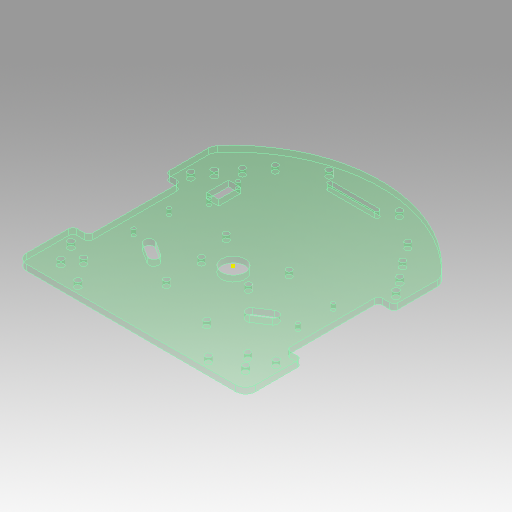
# Autodesk Inventor part: base_chasis_v6
Saved by Autodesk Inventor 2027 (Build 310192000, 192)
## iProperties
Created: 2025-03-12
Part Number: base_chasis_v6
Material: Generic
Document SubType Name: Modeling
Designer: cdavi
Density: 1 g/cm^3
Appearance: Clear - Green 1
Author: cdavi
Autodesk Inventor part; units mm, degrees
ref_plane "YZ Plane" through (0, 0, 0) normal (1, 0, 0) x (0, 1, 0)
ref_plane "XZ Plane" through (0, 0, 0) normal (0, 1, 0) x (-1, 0, 0)
ref_plane "XY Plane" through (0, 0, 0) normal (0, 0, 1) x (1, 0, 0)
sketch "Sketch1" plane through (0, 0, 0) normal (0, 1, 0) x (-1, 0, 0)
  line L0 (50.9902, 55) -> (-50.9902, 55)
  line L1 (12, -62.25) -> (-12, -62.25)
  line L2 (-12, -60) -> (12, -60)
  circle A0 centre (0, 0) radius 6
  circle A1 centre (-44.3523, -52.8571) radius 1.5 construction
  circle A2 centre (-41.7906, 34.5) radius 1.5
  circle A3 centre (-20, 51.5) radius 1.5 construction
  circle A4 centre (41.7906, 34.5) radius 1.5
  circle A5 centre (20, 51.5) radius 1.5 construction
  circle A6 centre (44.3523, -52.8571) radius 1.5 construction
  arc A7 (12, -62.25) -> (12, -60) centre (12, -61.125) ccw
  arc A8 (-12, -60) -> (-12, -62.25) centre (-12, -61.125) ccw
  circle A9 centre (0, 0) radius 69 construction
  line L3 (0, 0) -> (0, 55)
  arc A10 (-50.9902, 55) -> (50.9902, 55) centre (0, 0) ccw
  line L4 (0, 0) -> (-75, 0)
  line L5 (0, 0) -> (62.5352, -29.1607) construction
  line L6 (0, 0) -> (69, 0)
  line L7 (0, 0) -> (41.7906, 34.5) construction
  line L8 (50.2232, 23.5) -> (71.2232, 23.5)
  line L9 (71.2232, 23.5) -> (71.2232, -23.5)
  line L10 (71.2232, -23.5) -> (50.2232, -23.5)
  line L11 (50.2232, -23.5) -> (50.2232, 23.5)
  line L12 (50.2232, 23.5) -> (71.2232, -23.5) construction
  line L13 (71.2232, 23.5) -> (50.2232, -23.5) construction
  circle A11 centre (41.8232, -9) radius 1
  circle A12 centre (41.8232, 9) radius 1
  circle A13 centre (16, -12.35) radius 1.5
  circle A14 centre (33.75, -55) radius 1.5
  circle A15 centre (-16, -12.35) radius 1.5
  circle A16 centre (-33.75, -55) radius 1.5
  line L14 (-50.2232, 23.5) -> (-71.2232, 23.5)
  line L15 (-71.2232, 23.5) -> (-71.2232, -23.5)
  line L16 (-71.2232, -23.5) -> (-50.2232, -23.5)
  line L17 (-50.2232, -23.5) -> (-50.2232, 23.5)
  circle A17 centre (-41.8232, -9) radius 1
  circle A18 centre (-41.8232, 9) radius 1
  line L18 (39, -25.5) -> (33, -25.5)
  line L19 (33, -25.5) -> (33, -36.5)
  line L20 (33, -36.5) -> (39, -36.5)
  line L21 (39, -36.5) -> (39, -25.5)
  circle A19 centre (36, -38.5) radius 1
  line L22 (39, -31) -> (33, -31)
  circle A20 centre (36, -23.5) radius 1
  circle A21 centre (40.817, -45.3318) radius 1.5
  circle A22 centre (-41.7906, 34.5) radius 1.5
  circle A23 centre (-40.817, -45.3318) radius 1.5
  line L23 (41.7906, 34.5) -> (41.7906, 39.5)
  line L24 (41.7906, 39.5) -> (63.7554, 39.5) construction
  line L25 (0, 0) -> (44.3523, -52.8571) construction
  line L26 (40.817, -45.3318) -> (0, 0) construction
  line L27 (0, 0) -> (62.5352, 29.1607) construction
  circle A24 centre (12, 4.32) radius 1.5
  circle A25 centre (-12, 4.32) radius 1.5
  line L28 (33.2906, 29.5) -> (34.2906, 29.5)
  line L29 (36.2906, 27.5) -> (36.2906, 21.5)
  line L30 (34.2906, 19.5) -> (33.2906, 19.5)
  line L31 (31.2906, 21.5) -> (31.2906, 27.5)
  arc A26 (34.2906, 19.5) -> (36.2906, 21.5) centre (34.2906, 21.5) ccw
  arc A27 (31.2906, 21.5) -> (33.2906, 19.5) centre (33.2906, 21.5) ccw
  arc A28 (33.2906, 29.5) -> (31.2906, 27.5) centre (33.2906, 27.5) ccw
  arc A29 (36.2906, 27.5) -> (34.2906, 29.5) centre (34.2906, 27.5) ccw
  line L32 (0, 0) -> (-41.7906, 34.5) construction
  line L33 (-33.2906, 29.5) -> (-34.2906, 29.5)
  line L34 (-36.2906, 27.5) -> (-36.2906, 21.5)
  line L35 (-34.2906, 19.5) -> (-33.2906, 19.5)
  line L36 (-31.2906, 21.5) -> (-31.2906, 27.5)
  arc A30 (-36.2906, 21.5) -> (-34.2906, 19.5) centre (-34.2906, 21.5) ccw
  arc A31 (-33.2906, 19.5) -> (-31.2906, 21.5) centre (-33.2906, 21.5) ccw
  arc A32 (-31.2906, 27.5) -> (-33.2906, 29.5) centre (-33.2906, 27.5) ccw
  arc A33 (-34.2906, 29.5) -> (-36.2906, 27.5) centre (-34.2906, 27.5) ccw
  circle A34 centre (0, 0) radius 54.1913
  circle A35 centre (0, 0) radius 61 construction
  point P0 (-5.9883, -61.0615)
  point P1 (60.7232, 0)
  point P2 (0, 34.5)
  point P3 (36, -36.5)
  point P4 (50.9902, 55)
  point P5 (0, -6)
  point P6 (31.2906, 29.5)
  point P7 (31.2906, 19.5)
  point P8 (33.7906, 29.5)
  point P9 (-31.2906, 29.5)
  point P10 (-31.2906, 19.5)
  point P11 (-33.7906, 29.5)
  dimension "d12" = 12
  dimension "d287" = 0
  dimension "d398" = 108.3827
  dimension "d0" = 3
  dimension "d1" = 3
  dimension "d15" = 24
  dimension "d16" = 3
  dimension "d62" = 2.25
  dimension "d148" = 3.5
  dimension "d276" = 138
  dimension "d285" = 150
  dimension "d286" = 55
  dimension "d288" = 12
  dimension "d289" = 40
  dimension "d290" = 3.5
  dimension "d291" = 20
  dimension "d293" = 25
  dimension "d300" = 21
  dimension "d301" = 47
  dimension "d304" = 2
  dimension "d305" = 8.4
  dimension "d306" = 9
  dimension "d307" = 3
  dimension "d311" = 16
  dimension "d318" = 33.75
  dimension "d323" = 11
  dimension "d324" = 6
  dimension "d325" = 2
  dimension "d326" = 2
  dimension "d327" = 15
  dimension "d338" = 33
  dimension "d342" = 5
  dimension "d345" = 11
  dimension "d346" = 39.541
  dimension "d348" = 40
  dimension "d350" = 61
  dimension "d351" = 48
  dimension "d352" = 3
  dimension "d353" = 12.35
  dimension "d354" = 55
  dimension "d355" = 25
  dimension "d356" = 60
  dimension "d358" = 71.2232
  dimension "d371" = 3
  dimension "d372" = 12
  dimension "d373" = 4.32
  dimension "d393" = 5
  dimension "d394" = 10
  dimension "d395" = 5
  dimension "d396" = 2
  dimension "d397" = 8
  constraints: 75 end point, 33 centre point, 30 point on circle, 29 symmetric about line, 11 point on line, 11 tangent, 9 horizontal, 8 coincident, 8 midpoint, 7 parallel, 5 equal radius, 5 perpendicular, 3 vertical, 3 vertical alignment, 1 horizontal alignment, 33 other
  measures "d0" diameter of A4
  measures "d1" diameter of A5
  measures "d15" distance of L1.end L1.start
  measures "d16" diameter of A6
  measures "d62" distance between parallel lines of L1 L2
  measures "d148" distance from line of L0 A5.centre
  measures "d276" diameter of A9
  measures "d285" diameter of A10
  measures "d286" distance from line of L0 point (0, 0)
  measures "d288" horizontal distance of point (0, 0) A7.centre
  measures "d289" distance of A5.centre A3.centre
  measures "d290" distance from line of L0 A3.centre
  measures "d291" distance from line of L3 A5.centre
  measures "d293" angle of L6 L5
  measures "d300" distance of L9.end L10.end
  measures "d301" distance of L10.end L8.start
  measures "d304" diameter of A11
  measures "d305" distance from line of L11 A11.centre
  measures "d306" distance from line of L6 A11.centre
  measures "d307" diameter of A13
  measures "d311" horizontal distance of point (0, 0) A13.centre
  measures "d318" distance from line of L3 A14.centre
  measures "d323" distance of L18.end L19.end
  measures "d324" distance of L18.start L18.end
  measures "d325" distance from line of L10.end L18
  measures "d326" diameter of A19
  measures "d327" distance of A20.centre A19.centre
  measures "d338" distance between parallel lines of L3 L19
  measures "d342" distance of L7.end L23.end
  measures "d345" distance from line of L8 L7.end
  measures "d346" angle of L6 L7
  measures "d348" angle of L3 L25
  measures "d350" distance of L26.start L4.start
  measures "d351" angle of L6 L26
  measures "d352" diameter of A21
  measures "d353" vertical distance of point (0, 0) A13.centre
  measures "d354" distance from line of L6 A14.centre
  measures "d355" angle of L27 L6
  measures "d356" distance between parallel lines of L2 L4
  measures "d358" distance between parallel lines of L3 L15
  measures "d371" diameter of A24
  measures "d372" horizontal distance of A24.centre point (0, 0)
  measures "d373" vertical distance of point (0, 0) A24.centre
  measures "d393" distance between parallel lines of L31 L29
  measures "d394" distance of point (31.291, 19.5) point (31.291, 29.5)
  measures "d395" distance from line of L7.end L28
  measures "d396" radius of A26
  measures "d397" horizontal distance of L7.end point (33.791, 29.5)
extrude "Extrusion1" add sketch "Sketch1" along normal blind 3 contours A10 L8 L11 A34 A4 L3 L0 | L3 A34 A2 L17 L14 A10 L0 | A34 A4 L11 L6 A0 L3 | L3 A0 L4 L17 A34 A2 | A10 L16 L17 A34 L11 L10 | L6 L11 A34 L17 L4 A0
sketch "Sketch3" plane through (0, 3, 0) normal (0, 1, 0) x (1, 0, 0)
  line L0 (3, 0) -> (3, -20)
  circle A0 centre (-11, -23.1) radius 1.5
  line L1 (-50.9902, -55) -> (50.9902, -55) projected
  circle A1 centre (17, -30.6) radius 1.5
  point P0 (0, 0)
  point P1 (-51.2348, -50)
  dimension "d377" = 20
  dimension "d378" = 3
  dimension "d379" = 3
  dimension "d380" = 14
  dimension "d381" = 31.9
  dimension "d383" = 14
  dimension "d384" = 3
  dimension "d385" = 24.4
  constraints: 2 centre point, 2 end point, 1 vertical, 1 other
  measures "d377" distance of L0.start L0.end
  measures "d378" distance from line of point (0, 0) L0
  measures "d379" diameter of A0
  measures "d380" distance from line of L0 A0.centre
  measures "d383" distance from line of A1.centre L0
  measures "d384" diameter of A1
fillet "Fillet1" radius 2 1 edges at (71.2232, 1.5, 23.5)
fillet "Fillet2" radius 2 7 edges at (71.2232, 1.5, -23.5) (-71.2232, 1.5, -23.5) (-71.2232, 1.5, 23.5) (-50.2232, 1.5, -23.5) (-50.2232, 1.5, 23.5) (50.2232, 1.5, -23.5) (50.2232, 1.5, 23.5)
hole "Hole1" at (-11, 3, 23.1) at (17, 3, 30.6) direction (0, -1, 0) diameter 3 end through all
sketch "Sketch4" plane through (0, 3, 0) normal (0, 1, 0) x (1, 0, 0)
  line L0 (-50.2232, 21.5) -> (-50.2232, -21.5) projected
  line L1 (-115.8769, 106.6342) -> (-58.2232, 106.6342)
  line L2 (-58.2232, 106.6342) -> (-58.2232, -77.5521)
  line L3 (-58.2232, -77.5521) -> (-115.8769, -77.5521)
  line L4 (-115.8769, -77.5521) -> (-115.8769, 106.6342)
  line L5 (-50.2232, 0) -> (-58.2232, 0)
  point P0 (0, 0)
  dimension "d403" = 8
  constraints: 10 end point, 2 parallel, 2 perpendicular, 1 horizontal, 1 midpoint, 1 point on line
  measures "d403" distance of L5.start L5.end
extrude "Extrusion3" cut sketch "Sketch4" against normal blind 10
mirror "Mirror1" about plane through (0, 0, 0) normal (1, 0, 0) of "Extrusion3"
fillet "Fillet3" radius 2 4 edges at (-58.2232, 1.5, 23.5) (-58.2232, 1.5, -23.5) (58.2232, 1.5, -23.5) (58.2232, 1.5, 23.5)
sketch "Sketch5" plane through (0, 3, 0) normal (0, 1, 0) x (1, 0, 0)
  point P0 (0, 0)
fillet "Fillet5" [suppressed]
sketch "Sketch6" plane through (0, 3, 0) normal (0, 1, 0) x (1, 0, 0)
  point P0 (0, 0)
sketch "Sketch7" plane through (0, 3, 0) normal (0, 1, 0) x (1, 0, 0)
  arc A0 (58.2232, 47.2764) -> (-58.2232, 47.2764) centre (0, 0) ccw projected
  line L0 (-58.2232, 47.2764) -> (-58.2232, 0)
  line L1 (-58.2232, 0) -> (0, 0)
  line L2 (-58.2232, 0) -> (-58.2232, 23.5)
  line L3 (-56.2232, 23.5) -> (-52.2232, 23.5) projected
  constraints: 6 end point, 1 horizontal, 1 perpendicular, 1 point on line, 1 vertical
sketch "Sketch8" plane through (0, 3, 0) normal (0, 1, 0) x (1, 0, 0)
  line L0 (58.2232, 47.2764) -> (58.2232, 25.5) projected
  line L1 (58.2232, 47.2764) -> (58.2232, 23)
  point P0 (0, 0)
  constraints: 2 end point, 1 vertical
fillet "Fillet6" radius 5 2 edges at (-58.2232, 1.5, -47.2764) (58.2232, 1.5, -47.2764)
sketch "Sketch9" plane through (0, 3, 0) normal (0, 1, 0) x (1, 0, 0)
  arc A0 (50.9902, -55) -> (58.2232, -47.2764) centre (0, 0) ccw projected
  line L0 (50.9902, -55) -> (58.2232, -55)
  line L1 (58.2232, -55) -> (58.2232, -47.2764)
  circle A1 centre (0, 0) radius 6 projected
  arc A2 (50.9902, -55) -> (58.2232, -47.2764) centre (0, 0) ccw
  constraints: 4 end point, 2 point on circle, 1 centre point, 1 coincident, 1 horizontal, 1 perpendicular
extrude "Extrusion4" add sketch "Sketch9" against normal blind 3 contours A0 L1 L0
mirror "Mirror2" about plane through (0, 0, 0) normal (1, 0, 0) of "Extrusion4"
sketch "Sketch10" plane through (0, 3, 0) normal (0, 1, 0) x (1, 0, 0)
  point P0 (0, 0)
sketch "Sketch11" plane through (0, 3, 0) normal (0, 1, 0) x (1, 0, 0)
  line L0 (-58.2232, -55) -> (58.2232, -55) projected
  line L1 (58.2232, -25.5) -> (58.2232, -55) projected
  line L2 (-58.2232, -55) -> (58.2232, -55)
  line L3 (58.2232, -55) -> (58.2232, -52)
  line L4 (58.2232, -52) -> (-58.2232, -52)
  line L5 (-58.2232, -52) -> (-58.2232, -55)
  point P0 (0, 0)
  dimension "d410" = 3
  constraints: 8 end point, 2 parallel, 1 horizontal, 1 perpendicular, 1 point on line
  measures "d410" distance between parallel lines of L0 L4
extrude "Extrusion5" cut sketch "Sketch11" against normal blind 3
fillet "Fillet7" radius 5 2 edges at (58.2232, 1.5, 52) (-58.2232, 1.5, 52)
sketch "Sketch12" plane through (0, 3, 0) normal (0, 1, 0) x (1, 0, 0)
  point P0 (0, 0)
sketch "Sketch13" plane through (0, 3, 0) normal (0, 1, 0) x (1, 0, 0)
  circle A0 centre (-33.2232, -46) radius 1.6
  line L0 (-53.2232, -52) -> (53.2232, -52) projected
  line L1 (-58.2232, -47) -> (-58.2232, -25.5) projected
  line L2 (53.2232, -52) -> (-53.2232, -52) projected
  line L3 (0, -52) -> (0, 75)
  arc A1 (57.0249, 48.7151) -> (-57.0249, 48.7151) centre (0, 0) ccw projected
  circle A2 centre (-52.2232, -30.525) radius 1.6
  line L4 (0, 0) -> (-64.2535, 0)
  line L5 (0, 0) -> (-17.8585, 66.6489)
  circle A3 centre (0, 0) radius 69
  circle A4 centre (0, 0) radius 6 projected
  circle A5 centre (-17.8585, 66.6489) radius 1.6
  circle A6 centre (33.2232, -46) radius 1.6
  circle A7 centre (52.2232, -30.525) radius 1.6
  circle A8 centre (17.8585, 66.6489) radius 1.6
  line L6 (-58.2232, 45.4674) -> (-58.2232, 25.5) projected
  line L7 (-56.2232, 23.5) -> (-52.2232, 23.5) projected
  circle A9 centre (-52.2232, 30.525) radius 1.6
  circle A10 centre (52.2232, 30.525) radius 1.6
  circle A11 centre (-47.2235, 37.4674) radius 1.6
  circle A12 centre (-47.0232, -40.8) radius 1.6
  circle A13 centre (47.2235, 37.4674) radius 1.6
  circle A14 centre (47.0232, -40.8) radius 1.6
  line L8 (-52.2232, -23.5) -> (-56.2232, -23.5) projected
  point P0 (-54.2232, 23.5)
  dimension "d414" = 3.2
  dimension "d415" = 6
  dimension "d416" = 25
  dimension "d417" = 3.2
  dimension "d418" = 6
  dimension "d420" = 75
  dimension "d421" = 6
  dimension "d422" = 3.2
  dimension "d427" = 3.2
  dimension "d428" = 6
  dimension "d429" = 7.025
  dimension "d430" = 3.2
  dimension "d432" = 10.9998
  dimension "d433" = 3.2
  dimension "d434" = 11.2
  dimension "d435" = 11.2
  dimension "d436" = 13.9674
  dimension "d437" = 7.025
  constraints: 12 centre point, 6 end point, 6 symmetric about line, 2 midpoint, 1 coincident, 1 horizontal, 1 point on circle, 1 point on line, 1 vertical, 10 other
  measures "d414" diameter of A0
  measures "d415" distance from line of L0 A0.centre
  measures "d416" distance from line of L1 A0.centre
  measures "d417" diameter of A2
  measures "d418" distance from line of L1 A2.centre
  measures "d420" angle of L4 L5
  measures "d422" diameter of A5
  measures "d427" diameter of A9
  measures "d428" distance from line of L6 A9.centre
  measures "d429" distance from line of L7 A9.centre
  measures "d430" diameter of A11
  measures "d432" distance from line of L6 A11.centre
  measures "d433" diameter of A12
  measures "d434" distance from line of L2 A12.centre
  measures "d435" distance from line of L1 A12.centre
  measures "d436" distance from line of L7 A11.centre
  measures "d437" distance from line of L8 A2.centre
extrude "Extrusion6" cut sketch "Sketch13" against normal blind 3 contours A0 | A5 A3 | A3 L5 A5 | A8 A3 | A3 A8 | A3 A5 L5 | A2 | A6 | A7 | A9 | A10 | A11 | A12 | A13 | A14
sketch "Sketch14" plane through (0, 0, 0) normal (0, -1, 0) x (1, 0, 0)
  circle A0 centre (47.2235, -37.4674) radius 1.6 projected
  circle A1 centre (-52.2232, 30.525) radius 1.6 projected
  circle A2 centre (17.8585, -66.6489) radius 1.6 projected
  circle A3 centre (52.2232, 30.525) radius 1.6 projected
  circle A4 centre (52.2232, -30.525) radius 1.6 projected
  circle A5 centre (-47.2235, -37.4674) radius 1.6 projected
  circle A6 centre (47.0232, 40.8) radius 1.6 projected
  circle A7 centre (-33.2232, 46) radius 1.6 projected
  circle A8 centre (-17.8585, -66.6489) radius 1.6 projected
  circle A9 centre (33.2232, 46) radius 1.6 projected
  circle A10 centre (-52.2232, -30.525) radius 1.6 projected
  circle A11 centre (-47.0232, 40.8) radius 1.6 projected
  arc A12 (-53.2232, 52) -> (-58.2232, 47) centre (-53.2232, 47) ccw projected
  line L0 (-53.2232, 52) -> (53.2232, 52) projected
  arc A13 (58.2232, 47) -> (53.2232, 52) centre (53.2232, 47) ccw projected
  line L1 (58.2232, 47) -> (58.2232, 25.5) projected
  arc A14 (56.2232, 23.5) -> (58.2232, 25.5) centre (56.2232, 25.5) ccw projected
  line L2 (56.2232, 23.5) -> (52.2232, 23.5) projected
  arc A15 (52.2232, 23.5) -> (50.2232, 21.5) centre (52.2232, 21.5) ccw projected
  line L3 (50.2232, 21.5) -> (50.2232, -21.5) projected
  arc A16 (50.2232, -21.5) -> (52.2232, -23.5) centre (52.2232, -21.5) ccw projected
  line L4 (52.2232, -23.5) -> (56.2232, -23.5) projected
  arc A17 (58.2232, -25.5) -> (56.2232, -23.5) centre (56.2232, -25.5) ccw projected
  line L5 (58.2232, -25.5) -> (58.2232, -45.4674) projected
  arc A18 (57.0249, -48.7151) -> (58.2232, -45.4674) centre (53.2232, -45.4674) ccw projected
  arc A19 (-57.0249, -48.7151) -> (57.0249, -48.7151) centre (0, 0) ccw projected
  arc A20 (-58.2232, -45.4674) -> (-57.0249, -48.7151) centre (-53.2232, -45.4674) ccw projected
  line L6 (-58.2232, -45.4674) -> (-58.2232, -25.5) projected
  arc A21 (-56.2232, -23.5) -> (-58.2232, -25.5) centre (-56.2232, -25.5) ccw projected
  line L7 (-56.2232, -23.5) -> (-52.2232, -23.5) projected
  arc A22 (-52.2232, -23.5) -> (-50.2232, -21.5) centre (-52.2232, -21.5) ccw projected
  line L8 (-50.2232, -21.5) -> (-50.2232, 21.5) projected
  arc A23 (-50.2232, 21.5) -> (-52.2232, 23.5) centre (-52.2232, 21.5) ccw projected
  line L9 (-52.2232, 23.5) -> (-56.2232, 23.5) projected
  arc A24 (-58.2232, 25.5) -> (-56.2232, 23.5) centre (-56.2232, 25.5) ccw projected
  line L10 (-58.2232, 25.5) -> (-58.2232, 47) projected
  circle A25 centre (17, 30.6) radius 1.5 projected
  circle A26 centre (-11, 23.1) radius 1.5 projected
  circle A27 centre (0, 0) radius 6 projected
  line L11 (12, -60) -> (-12, -60) projected
  arc A28 (-12, -60) -> (-12, -62.25) centre (-12, -61.125) ccw projected
  line L12 (-12, -62.25) -> (12, -62.25) projected
  arc A29 (12, -62.25) -> (12, -60) centre (12, -61.125) ccw projected
  circle A30 centre (-41.8232, -9) radius 1 projected
  circle A31 centre (-16, -12.35) radius 1.5 projected
  circle A32 centre (-33.75, -55) radius 1.5 projected
  circle A33 centre (16, -12.35) radius 1.5 projected
  circle A34 centre (33.75, -55) radius 1.5 projected
  circle A35 centre (41.8232, -9) radius 1 projected
  circle A36 centre (-36, -38.5) radius 1 projected
  circle A37 centre (-36, -23.5) radius 1 projected
  circle A38 centre (-40.817, -45.3318) radius 1.5 projected
  circle A39 centre (40.817, -45.3318) radius 1.5 projected
  line L13 (-33, -25.5) -> (-39, -25.5) projected
  line L14 (-39, -25.5) -> (-39, -36.5) projected
  line L15 (-39, -36.5) -> (-33, -36.5) projected
  line L16 (-33, -36.5) -> (-33, -25.5) projected
  circle A40 centre (41.8232, 9) radius 1 projected
  circle A41 centre (12, 4.32) radius 1.5 projected
  arc A42 (34.2906, 19.5) -> (36.2906, 21.5) centre (34.2906, 21.5) ccw projected
  line L17 (36.2906, 21.5) -> (36.2906, 27.5) projected
  arc A43 (36.2906, 27.5) -> (34.2906, 29.5) centre (34.2906, 27.5) ccw projected
  line L18 (34.2906, 29.5) -> (33.2906, 29.5) projected
  arc A44 (33.2906, 29.5) -> (31.2906, 27.5) centre (33.2906, 27.5) ccw projected
  line L19 (31.2906, 27.5) -> (31.2906, 21.5) projected
  arc A45 (31.2906, 21.5) -> (33.2906, 19.5) centre (33.2906, 21.5) ccw projected
  line L20 (33.2906, 19.5) -> (34.2906, 19.5) projected
  circle A46 centre (41.7906, 34.5) radius 1.5 projected
  circle A47 centre (-41.7906, 34.5) radius 1.5 projected
  line L21 (-31.2906, 21.5) -> (-31.2906, 27.5) projected
  arc A48 (-31.2906, 27.5) -> (-33.2906, 29.5) centre (-33.2906, 27.5) ccw projected
  line L22 (-33.2906, 29.5) -> (-34.2906, 29.5) projected
  arc A49 (-34.2906, 29.5) -> (-36.2906, 27.5) centre (-34.2906, 27.5) ccw projected
  line L23 (-36.2906, 27.5) -> (-36.2906, 21.5) projected
  arc A50 (-36.2906, 21.5) -> (-34.2906, 19.5) centre (-34.2906, 21.5) ccw projected
  line L24 (-34.2906, 19.5) -> (-33.2906, 19.5) projected
  arc A51 (-33.2906, 19.5) -> (-31.2906, 21.5) centre (-33.2906, 21.5) ccw projected
  circle A52 centre (-12, 4.32) radius 1.5 projected
  circle A53 centre (-41.8232, 9) radius 1 projected
  line L25 (-36.2906, 21.5) -> (-36.2906, 27.5)
  arc A54 (-34.2906, 29.5) -> (-36.2906, 27.5) centre (-34.2906, 27.5) ccw
  line L26 (-34.2906, 29.5) -> (-33.2906, 29.5)
  arc A55 (-31.2906, 27.5) -> (-33.2906, 29.5) centre (-33.2906, 27.5) ccw
  line L27 (-31.2906, 27.5) -> (-31.2906, 21.5)
  arc A56 (-33.2906, 19.5) -> (-31.2906, 21.5) centre (-33.2906, 21.5) ccw
  line L28 (-33.2906, 19.5) -> (-34.2906, 19.5)
  arc A57 (-36.2906, 21.5) -> (-34.2906, 19.5) centre (-34.2906, 21.5) ccw
  line L29 (31.2906, 21.5) -> (31.2906, 27.5)
  arc A58 (33.2906, 29.5) -> (31.2906, 27.5) centre (33.2906, 27.5) ccw
  line L30 (33.2906, 29.5) -> (34.2906, 29.5)
  arc A59 (36.2906, 27.5) -> (34.2906, 29.5) centre (34.2906, 27.5) ccw
  line L31 (36.2906, 27.5) -> (36.2906, 21.5)
  arc A60 (34.2906, 19.5) -> (36.2906, 21.5) centre (34.2906, 21.5) ccw
  line L32 (34.2906, 19.5) -> (33.2906, 19.5)
  arc A61 (31.2906, 21.5) -> (33.2906, 19.5) centre (33.2906, 21.5) ccw
  point P0 (-36.2906, 24.5)
  point P1 (-36.2906, 24.5)
  dimension "d438" = 0
  dimension "d439" = 0
  constraints: 16 end point, 16 point on circle, 8 centre point, 2 midpoint, 14 other
  measures "d438" distance of point (-36.291, 24.5) point (-36.291, 24.5)
  measures "d439" distance between parallel lines of L29 L19
extrude "Extrusion7" add sketch "Sketch14" against normal blind 3 contours L20 A45 L19 A44 L18 A43 L17 A42 | A51 L24 A50 L23 A49 L22 A48 L21
sketch "Sketch15" plane through (0, 0, 0) normal (0, -1, 0) x (1, 0, 0)
  circle A0 centre (-41.7906, 34.5) radius 1.5 projected
  circle A1 centre (-41.7906, 34.5) radius 1.5
  line L0 (-41.7906, 34.5) -> (-40.2906, 34.5)
  line L1 (-41.7906, 34.5) -> (-32.5514, 40.5)
  line L2 (-31.6746, 11.2603) -> (-24.6746, 15.8062) construction
  line L3 (-30.313, 9.1636) -> (-23.313, 13.7095)
  line L4 (-26.0362, 17.9028) -> (-33.0362, 13.357)
  arc A2 (-33.0362, 13.357) -> (-30.313, 9.1636) centre (-31.6746, 11.2603) ccw
  arc A3 (-23.313, 13.7095) -> (-26.0362, 17.9028) centre (-24.6746, 15.8062) ccw
  line L5 (-41.7906, 34.5) -> (-26.813, 11.4366)
  point P0 (0, 0)
  point P1 (-28.1746, 13.5332)
  dimension "d446" = 6
  dimension "d447" = 33
  dimension "d448" = 25
  dimension "d449" = 5
  dimension "d450" = 7
  constraints: 14 end point, 4 point on circle, 4 tangent, 2 centre point, 2 midpoint, 2 parallel, 2 point on line, 1 coincident, 1 horizontal, 1 horizontal alignment, 1 perpendicular, 3 other
  measures "d446" vertical distance of L0.start L1.end
  measures "d447" angle of L0 L1
  measures "d448" distance between parallel lines of L1 L2
  measures "d449" distance between parallel lines of L3 L4
  measures "d450" horizontal distance of L2.end L2.start
extrude "Extrusion8" cut sketch "Sketch15" against normal blind 3 contours A2 L4 L5 L3 | L5 L4 A3 L3
mirror "Mirror3" about plane through (0, 0, 0) normal (1, 0, 0) of "Extrusion8"
body "Solid1"
